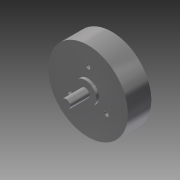
# Autodesk Inventor part: Moteur MAxon
Saved by Autodesk Inventor 2014 SP2 (Build 180246200, 246)
## iProperties
Created: 2015-09-22
Part Number: Moteur MAxon
Material: Acier inoxydable
Document SubType Name: Modeling
Designer: sd
Density: 8.08 g/cm^3
Appearance: Semi-poli
Mass: 1449.9 g
Surface Area: 218.077 cm^2
Volume: 179.444 cm^3
Author: sd
Autodesk Inventor part; units mm, degrees
ref_plane "YZ Plane" through (0, 0, 0) normal (1, 0, 0) x (0, 1, 0)
ref_plane "XZ Plane" through (0, 0, 0) normal (0, 1, 0) x (-1, 0, 0)
ref_plane "XY Plane" through (0, 0, 0) normal (0, 0, 1) x (1, 0, 0)
sketch "Esquisse1" plane through (0, 0, 0) normal (0, 1, 0) x (-1, 0, 0)
  circle A0 centre (0, 0) radius 45
  dimension "d0" = 90
  constraints: 1 centre point, 1 coincident
  measures "d0" diameter of A0
extrude "Extrusion1" add sketch "Esquisse1" along normal blind 27.3
fillet "Congé1" radius 1 1 edges at (45, 27.3, 0)
sketch "Esquisse2" plane through (0, 27.3, 0) normal (0, 1, 0) x (1, 0, 0)
  circle A0 centre (0, 0) radius 44 projected
  circle A1 centre (0, 0) radius 20
  dimension "d4" = 40
  constraints: 1 centre point, 1 coincident
  measures "d4" diameter of A1
extrude "Extrusion2" add sketch "Esquisse2" along normal blind 2.3 contours A1
fillet "Congé2" radius 0.5 1 edges at (-20, 29.6, 0)
sketch "Esquisse3" plane through (0, 0, 0) normal (0, -1, 0) x (1, 0, 0)
  circle A0 centre (0, 0) radius 45 projected
  circle A1 centre (0, 0) radius 12.5
  dimension "d8" = 25
  constraints: 1 centre point, 1 coincident
  measures "d8" diameter of A1
extrude "Extrusion3" add sketch "Esquisse3" along normal blind 3.2 contours A1
sketch "Esquisse5" plane through (0, -3.2, 0) normal (0, -1, 0) x (1, 0, 0)
  circle A0 centre (0, 0) radius 12.5 projected
  circle A1 centre (0, 0) radius 5
  dimension "d11" = 10
  constraints: 1 centre point, 1 coincident
  measures "d11" diameter of A1
extrude "Extrusion4" add sketch "Esquisse5" along normal blind 22 contours A1
sketch "Esquisse6" plane through (0, 0, 0) normal (0, -1, 0) x (1, 0, 0)
  circle A0 centre (0, 0) radius 12.5 projected
  circle A1 centre (0, 24) radius 2.5
  dimension "d14" = 5
  dimension "d15" = 24
  constraints: 1 centre point
  measures "d14" diameter of A1
  measures "d15" distance of A0.centre A1.centre
extrude "Extrusion5" cut sketch "Esquisse6" against normal blind 6 contours A1
pattern_circular "Réseau circulaire1" count 3 over 360 about axis through (0, 0, 0) along (0, -1, 0) of "Extrusion5"
